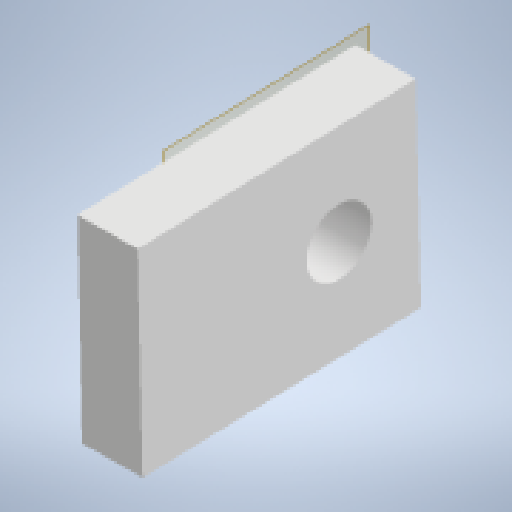
# Autodesk Inventor part: хвост
Saved by Autodesk Inventor 2024.2 (Build 282272000, 272)
## iProperties
Created: 2026-04-03
Part Number: хвост
Material: Типовые
Document SubType Name: Modeling
Designer: katya_notebook
Density: 1 g/cm^3
Appearance: По умолчанию
Author: katya_notebook
Autodesk Inventor part; units mm, degrees
ref_plane "YZ Plane" through (0, 0, 0) normal (1, 0, 0) x (0, 1, 0)
ref_plane "XZ Plane" through (0, 0, 0) normal (0, 1, 0) x (-1, 0, 0)
ref_plane "XY Plane" through (0, 0, 0) normal (0, 0, 1) x (1, 0, 0)
ref_plane "РабПлоскость1" through (-185.8888, -38.5334, 331.0061) normal (0.9999756, 0.0023998, -0.0065586) x (-0.0066118, 0.0228778, -0.9997164)
sketch "Эскиз9" plane through (-185.8888, -38.5334, 331.0061) normal (0.9999756, 0.0023998, -0.0065586) x (-0.0066118, 0.0228778, -0.9997164)
  circle A0 centre (-0.0036, 0) radius 3.25 projected
  line L0 (7.9964, 10) -> (7.9964, -10) projected
  line L1 (7.9964, 10) -> (-0.0036, 10) projected
  arc A1 (-0.0036, 10) -> (-0.0036, -10) centre (-0.0036, 0) ccw projected
  line L2 (-0.0036, -10) -> (7.9964, -10) projected
  line L3 (-0.0036, 10) -> (-20.0036, 10)
  line L4 (-0.0036, -10) -> (-20.0036, -10)
  line L5 (-20.0036, 10) -> (-20.0036, -10)
  point P0 (330.5647, 30.5274)
  dimension "d24" = 20
  constraints: 6 end point, 2 horizontal, 1 perpendicular
  measures "d24" distance of L1.end L3.end
extrude "Выдавливание4" add sketch "Эскиз9" along normal blind 6
